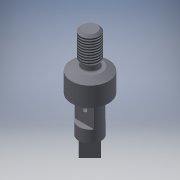
# Autodesk Inventor part: Вал 1
Saved by Autodesk Inventor 2016 (Build 200138000, 138)
## iProperties
Created: 2016-10-21
Part Number: Вал 1
Document SubType Name: Modeling
Density: 7.85 g/cm^3
Material: Сталь
Mass: 456.668 g
Surface Area: 117.348 cm^2
Volume: 58.1742 cm^3
Appearance: Сталь
Autodesk Inventor part; units mm, degrees
ref_plane "YZ Plane" through (0, 0, 0) normal (1, 0, 0) x (0, 1, 0)
ref_plane "XZ Plane" through (0, 0, 0) normal (0, 1, 0) x (-1, 0, 0)
sketch "Эскиз2" plane through (0, 0, 0) normal (0, 0, 1) x (1, 0, 0)
  line L0 (0.0208, 12) -> (12, 0.0208)
  line L1 (12, -0.0208) -> (0.0208, -12)
  line L2 (-0.0208, -12) -> (-12, -0.0208)
  line L3 (-12, 0.0208) -> (-0.0208, 12)
  circle A0 centre (0, 0) radius 12
  dimension "d4" = 24
  dimension "d0" = 17
  constraints: 8 end point, 2 coincident, 15 other
  measures "d0" distance between parallel lines of L1 L3
extrude "Выдавливание1" add sketch "Эскиз2" along normal blind 55
extrude "Выдавливание2" cut sketch "Эскиз2" along normal blind 16 contours A0 L0 | L3 A0 | A0 L1 | L2 A0
ref_plane "РабПлоскость1" through (0, 0, 49) normal (0, 0, 1) x (1, 0, 0)
sketch "Эскиз6" plane through (0, 0, 49) normal (0, 0, 1) x (1, 0, 0)
  line L0 (-26.028, 20.7085) -> (26.3443, 20.7085)
  line L1 (26.3443, 20.7085) -> (26.3443, 6)
  line L2 (26.3443, 6) -> (-26.028, 6)
  line L3 (-26.028, 6) -> (-26.028, 20.7085)
  point P0 (0, 0)
  dimension "d10" = 6
  constraints: 8 end point, 2 parallel, 1 horizontal, 1 perpendicular
  measures "d10" distance from line of point (0, 0) L2
extrude "Выдавливание3" cut sketch "Эскиз6" against normal blind 20
mirror "Зеркальное отражение1" about plane through (0, 0, 0) normal (0, 1, 0) of "Выдавливание3"
sketch "Эскиз7" plane through (0, 0, 0) normal (0, 1, 0) x (-1, 0, 0)
  line L0 (-12, 55) -> (12, 55) projected
  circle A0 centre (0, 43) radius 3
  point P0 (0, 0)
  dimension "d13" = 12
  dimension "d21" = 6
  constraints: 1 centre point, 1 coincident
  measures "d13" distance from line of point (0, 43) L0
  measures "d21" diameter of A0
extrude "Выдавливание4" cut sketch "Эскиз7" along normal through all both and the other way through all
sketch "Эскиз8" plane through (0, 0, 55) normal (0, 0, 1) x (1, 0, 0)
  circle A0 centre (0, 0) radius 12 projected
  circle A1 centre (0, 0) radius 20
  dimension "d24" = 40
  constraints: 1 centre point, 1 coincident
  measures "d24" diameter of A1
extrude "Выдавливание5" add sketch "Эскиз8" along normal blind 25 contours A0 | A1
chamfer "Фаска1" distance 7.5 distance2 4.3301 1 edges at (-20, 0, 80) measured on face at (-19.5, 0, 80)
sketch "Эскиз9" plane through (0, 0, 80) normal (0, 0, 1) x (1, 0, 0)
  circle A0 centre (0, 0) radius 12.5 projected
  circle A1 centre (0, 0) radius 8.25
  dimension "d30" = 16.5
  constraints: 1 centre point, 1 coincident
  measures "d30" diameter of A1
extrude "Выдавливание6" add sketch "Эскиз9" along normal blind 6 contours A1
sketch "Эскиз10" plane through (0, 0, 86) normal (0, 0, 1) x (1, 0, 0)
  circle A0 centre (0, 0) radius 8.25 projected
  circle A1 centre (0, 0) radius 10
  dimension "d33" = 20
  constraints: 1 centre point, 1 coincident
  measures "d33" diameter of A1
extrude "Выдавливание7" add sketch "Эскиз10" along normal blind 29 contours A0 | A1
thread "Резьба1" size "M20x2.5" class "6g" standard "ANSI Metric M Profile" full length
chamfer "Фаска2" distance 1.75 angle 45 1 edges at (-10, 0, 86) measured on face at (-9.5, 0, 86)
chamfer "Фаска3" distance 2.5 angle 45 1 edges at (-10, 0, 115) measured on face at (-9.5, 0, 115)
fillet "Сопряжение1" radius 1.6 1 edges at (-8.25, 0, 80)
fillet "Сопряжение2" radius 1 2 edges at (-8.25, 0, 86) (-8.2501, 0, 86)
